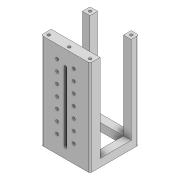
# Autodesk Inventor part: 00_Linear_Stage_NEMA11_Mount
Saved by Autodesk Inventor 2022 (Build 260153000, 153)
## iProperties
Created: 2022-02-11
Part Number: 00_Linear_Stage_NEMA11_Mount
Material: Generic
Document SubType Name: Modeling
Designer: wanghaoran
Density: 1 g/cm^3
Appearance: Default
Author: wanghaoran
Autodesk Inventor part; units mm, degrees
ref_plane "YZ Plane" through (0, 0, 0) normal (1, 0, 0) x (0, 1, 0)
ref_plane "XZ Plane" through (0, 0, 0) normal (0, 1, 0) x (-1, 0, 0)
ref_plane "XY Plane" through (0, 0, 0) normal (0, 0, 1) x (1, 0, 0)
sketch "Sketch1" plane through (0, 0, 0) normal (0, 1, 0) x (-1, 0, 0)
  line L0 (0, 0) -> (49.8, 0)
  line L1 (49.8, 0) -> (49.8, -49.8)
  line L2 (49.8, -49.8) -> (0, -49.8)
  line L3 (0, -49.8) -> (0, 0)
  line L4 (7.8, -7.8) -> (42, -7.8)
  line L5 (42, -7.8) -> (42, -42)
  line L6 (42, -42) -> (7.8, -42)
  line L7 (7.8, -42) -> (7.8, -7.8)
  dimension "d0" = 49.8
  dimension "d1" = 49.8
  dimension "d2" = 7.8
  constraints: 16 end point, 4 parallel, 2 perpendicular, 1 horizontal, 3 other
  measures "d0" distance of L1.end L2.end
  measures "d1" distance of L0.end L1.end
  measures "d2" distance between parallel lines of L3 L7
extrude "Extrusion1" add sketch "Sketch1" along normal blind 8
sketch "Sketch3" plane through (0, 0, 0) normal (0, -1, 0) x (1, 0, 0)
  line L0 (-49.8, 0) -> (0, 0) projected
  line L1 (-49.8, -49.8) -> (-49.8, 0) projected
  line L2 (0, 0) -> (-49.8, 0)
  line L3 (-49.8, 0) -> (-49.8, -10.23)
  line L4 (-49.8, -10.23) -> (0, -10.23)
  line L5 (0, -10.23) -> (0, 0)
  line L6 (-7.8, -42) -> (-7.8, -7.8) projected
  line L7 (0, -49.8) -> (-7.8, -49.8)
  line L8 (-7.8, -49.8) -> (-7.8, -42)
  line L9 (-7.8, -42) -> (0, -42)
  line L10 (0, -42) -> (0, -49.8)
  line L11 (0, -49.8) -> (-49.8, -49.8) projected
  line L12 (-42, -7.8) -> (-42, -42) projected
  line L13 (-49.8, -49.8) -> (-42, -49.8)
  line L14 (-42, -49.8) -> (-42, -42)
  line L15 (-42, -42) -> (-49.8, -42)
  line L16 (-49.8, -42) -> (-49.8, -49.8)
  dimension "d6" = 10.23
  constraints: 24 end point, 6 parallel, 3 horizontal, 3 perpendicular, 1 point on line
  measures "d6" distance of L3.end L2.end
extrude "Extrusion2" add sketch "Sketch3" against normal blind 97 contours L0 L5 L4 L1 | L15 L14 L11 L1 | L9 L10 L7 L8
sketch "Sketch4" plane through (-49.8, 0, 0) normal (0, 0, 1) x (1, 0, 0)
  line L0 (23.45, 81) -> (26.35, 81)
  line L1 (26.35, 81) -> (26.35, 11)
  line L2 (26.35, 11) -> (23.45, 11)
  line L3 (23.45, 11) -> (23.45, 81)
  line L4 (49.8, 0) -> (49.8, 97) projected
  line L5 (0, 0) -> (49.8, 0) projected
  circle A0 centre (24.9, 81) radius 1.45
  circle A1 centre (24.9, 11) radius 1.45
  circle A2 centre (16.4, 84) radius 1.45
  circle A3 centre (33.4, 84) radius 1.45
  line L6 (0, 97) -> (49.8, 97) projected
  circle A4 centre (16.4, 73) radius 1.45
  circle A5 centre (33.4, 73) radius 1.45
  circle A6 centre (16.4, 62) radius 1.45
  circle A7 centre (33.4, 62) radius 1.45
  circle A8 centre (16.4, 51) radius 1.45
  circle A9 centre (33.4, 51) radius 1.45
  circle A10 centre (16.4, 40) radius 1.45
  circle A11 centre (33.4, 40) radius 1.45
  circle A12 centre (16.4, 29) radius 1.45
  circle A13 centre (33.4, 29) radius 1.45
  circle A14 centre (16.4, 18) radius 1.45
  circle A15 centre (33.4, 18) radius 1.45
  dimension "d9" = 2.9
  dimension "d10" = 70
  dimension "d11" = 23.45
  dimension "d12" = 11
  dimension "d15" = 2.9
  dimension "d16" = 7.05
  dimension "d17" = 2.9
  dimension "d18" = 7.05
  dimension "d19" = 13
  dimension "d20" = 13
  dimension "d23" = 11
  constraints: 14 centre point, 8 end point, 2 midpoint, 2 parallel, 1 horizontal, 1 perpendicular, 1 vertical, 30 other
  measures "d9" distance of L1.end L2.end
  measures "d10" distance of L0.end L1.end
  measures "d11" distance between parallel lines of L4 L1
  measures "d12" distance between parallel lines of L5 L2
  measures "d15" diameter of A2
  measures "d16" distance from line of L3 A2.centre
  measures "d17" diameter of A3
  measures "d18" distance from line of A3.centre L1
  measures "d19" distance from line of L6 A2.centre
  measures "d20" distance from line of L6 A3.centre
  measures "d23" distance of A2.centre A4.centre
extrude "Extrusion3" cut sketch "Sketch4" against normal through all
sketch "Sketch5" plane through (0, 97, 0) normal (0, 1, 0) x (1, 0, 0)
  circle A0 centre (-45.9, 45.9) radius 1.4
  circle A1 centre (-3.9, 45.9) radius 1.4
  line L0 (-49.8, 49.8) -> (-49.8, 0) projected
  line L1 (-49.8, 24.9) -> (-42, 24.9)
  line L2 (-42, 10.23) -> (-42, 42) projected
  circle A2 centre (-45.9, 3.9) radius 1.4
  circle A3 centre (-3.9, 3.9) radius 1.4
  point P0 (0, 0)
  dimension "d28" = 2.8
  dimension "d29" = 2.8
  constraints: 4 centre point, 2 end point, 2 symmetric about line, 1 horizontal, 1 midpoint, 1 point on line, 2 other
  measures "d28" diameter of A0
  measures "d29" diameter of A1
extrude "Extrusion4" cut sketch "Sketch5" against normal blind 20
sketch "Sketch6" plane through (0, 0, 0) normal (0, -1, 0) x (1, 0, 0)
  line L0 (-49.8, 0) -> (0, 0) projected
  circle A0 centre (-24.9, -3.7) radius 1.4
  line L1 (-49.8, -49.8) -> (-49.8, 0) projected
  dimension "d37" = 2.8
  dimension "d38" = 3.7
  dimension "d39" = 24.9
  constraints: 1 centre point
  measures "d37" diameter of A0
  measures "d38" distance from line of L0 A0.centre
  measures "d39" distance from line of L1 A0.centre
extrude "Extrusion5" cut sketch "Sketch6" against normal blind 10
fillet "Fillet1" radius 2 4 edges at (0, 48.5, 0) (0, 48.5, -49.8) (-49.8, 48.5, -49.8) (-49.8, 48.5, 0)
sketch "Sketch7" plane through (0, 97, 0) normal (0, 1, 0) x (1, 0, 0)
  circle A0 centre (-24.9, 3.7) radius 1.4 projected
  circle A1 centre (-24.9, 3.7) radius 1.4
  point P0 (0, 0)
  constraints: 1 centre point, 1 coincident
extrude "Extrusion6" cut sketch "Sketch7" against normal blind 10
body "Solid1"
